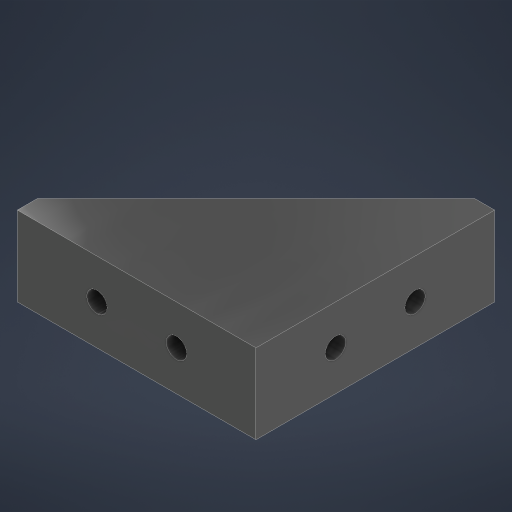
# Autodesk Inventor part: STRU_017_AngleBRacket_90_Plastic
Saved by Autodesk Inventor 2024.2 (Build 282272000, 272)
## iProperties
Created: 2024-07-25
Part Number: STRU_017_AngleBRacket_90_Plastic
Material: ABS Plastic
Document SubType Name: Modeling
Designer: Bryan
Density: 1.06 g/cm^3
Appearance: Dark Gray
Author: Bryan
Autodesk Inventor part; units mm, degrees
ref_plane "YZ Plane" through (0, 0, 0) normal (1, 0, 0) x (0, 1, 0)
ref_plane "XZ Plane" through (0, 0, 0) normal (0, 1, 0) x (-1, 0, 0)
ref_plane "XY Plane" through (0, 0, 0) normal (0, 0, 1) x (1, 0, 0)
sketch "Sketch1" plane through (0, 0, 0) normal (0, 1, 0) x (-1, 0, 0)
  line L0 (0, 0) -> (76.2, 0)
  line L1 (76.2, 0) -> (76.2, -6.35)
  line L2 (76.2, -6.35) -> (6.35, -6.35)
  line L3 (6.35, -6.35) -> (6.35, -76.2)
  line L4 (6.35, -76.2) -> (0, -76.2)
  line L5 (0, -76.2) -> (0, 0)
  dimension "d0" = 6.35
  dimension "d1" = 6.35
  dimension "d2" = 76.2
  dimension "d3" = 76.2
  constraints: 12 end point, 3 horizontal, 3 vertical
  measures "d0" distance between parallel lines of L2 L0
  measures "d1" distance of L3.end L4.end
  measures "d2" distance of L4.end L0.start
  measures "d3" distance of L0.start L0.end
extrude "Extrusion1" add sketch "Sketch1" along normal blind 25.4
sketch "Sketch2" plane through (0, 0, 0) normal (1, 0, 0) x (0, 0, -1)
  line L0 (0, 0) -> (0, 25.4) construction
  line L1 (0, 12.7) -> (76.2, 12.7) construction
  line L2 (76.2, 0) -> (76.2, 25.4) construction
  circle A0 centre (25.4, 12.7) radius 3.2512
  circle A1 centre (50.8, 12.7) radius 3.2512
  line L3 (0, 0) -> (0, 25.4) projected
  dimension "d6" = 6.5024
  dimension "d7" = 25.4
  dimension "d8" = 25.4
  constraints: 3 midpoint, 2 centre point, 2 end point, 2 point on line, 1 equal radius
  measures "d6" diameter of A0
  measures "d7" distance of A1.centre A0.centre
  measures "d8" distance of point (0, 12.7) A0.centre
extrude "Extrusion2" cut sketch "Sketch2" against normal blind 25.4
sketch "Sketch3" plane through (-76.2, 0, 0) normal (0, 0, 1) x (1, 0, 0)
  line L0 (0, 0) -> (0, 25.4) construction
  line L1 (0, 12.7) -> (76.2, 12.7) construction
  line L2 (76.2, 0) -> (76.2, 25.4) construction
  circle A0 centre (25.4, 12.7) radius 3.2512
  circle A1 centre (50.8, 12.7) radius 3.2512
  dimension "d11" = 6.5024
  dimension "d12" = 25.4
  dimension "d13" = 25.4
  constraints: 2 centre point, 2 end point, 2 midpoint, 2 point on line, 1 equal radius
  measures "d11" diameter of A0
  measures "d12" distance from line of L0 A0.centre
  measures "d13" distance of A1.centre A0.centre
extrude "Extrusion3" cut sketch "Sketch3" against normal blind 25.4
sketch "Sketch5" plane through (-6.35, 0, -6.35) normal (0, 0, -1) x (-1, 0, 0)
  line L0 (-6.35, 0) -> (0, 0) projected
  line L1 (69.85, 0) -> (69.85, 25.4) projected
  line L2 (0, 0) -> (69.85, 0)
  line L3 (69.85, 0) -> (69.85, 3.175)
  line L4 (69.85, 3.175) -> (0, 3.175)
  line L5 (0, 3.175) -> (0, 0)
  line L6 (69.85, 25.4) -> (0, 25.4)
  line L7 (0, 25.4) -> (0, 22.225)
  line L8 (0, 22.225) -> (69.85, 22.225)
  line L9 (69.85, 22.225) -> (69.85, 25.4)
  dimension "d18" = 3.175
  dimension "d19" = 3.175
  constraints: 16 end point, 4 parallel, 2 horizontal, 2 perpendicular, 2 point on line
  measures "d18" distance of L3.end L2.end
  measures "d19" distance of L7.end L6.end
sketch "Sketch4" plane through (-6.35, 0, -76.2) normal (-1, 0, 0) x (0, 0, 1)
  line L0 (69.85, 0) -> (69.85, 25.4) projected
  line L1 (0, 0) -> (69.85, 0)
  line L2 (69.85, 0) -> (69.85, 3.175)
  line L3 (69.85, 3.175) -> (0, 3.175)
  line L4 (0, 3.175) -> (0, 0)
  line L5 (0, 25.4) -> (69.85, 25.4) projected
  line L6 (0, 25.4) -> (69.85, 25.4)
  line L7 (69.85, 25.4) -> (69.85, 22.225)
  line L8 (69.85, 22.225) -> (0, 22.225)
  line L9 (0, 22.225) -> (0, 25.4)
  point P0 (76.2, 0)
  dimension "d16" = 3.175
  dimension "d17" = 3.175
  constraints: 16 end point, 4 parallel, 2 horizontal, 2 perpendicular, 2 point on line
  measures "d16" distance of L2.end L1.end
  measures "d17" distance of L6.end L7.end
loft "Loft1" add profiles "Sketch4", "Sketch5" contours L1 L4 L3 L0 / L2 L5 L4 L1
loft "Loft2" add profiles "Sketch4", "Sketch5" contours L8 L9 L5 L0 / L8 L7 L6 L1
body "Solid1"
